Autodesk Inventor part; units mm, degrees
(part 2 of 3)
  line L885 (90.7927, 5.4708) -> (90.7927, 2.3716)
  line L886 (90.7927, 2.3716) -> (91.5937, 2.3716)
  line L887 (91.5937, 2.3716) -> (91.5937, 1.3712)
  line L888 (91.5937, 1.3712) -> (105.5927, 1.3712)
  line L889 (105.5927, 1.3712) -> (105.5927, 2.3716)
  line L890 (105.5927, 2.3716) -> (106.3937, 2.3716)
  line L891 (106.3937, 2.3716) -> (106.3937, 5.4708)
  line L892 (106.3937, 5.4708) -> (105.5927, 5.4708)
  line L893 (105.5927, 5.4708) -> (105.5927, 11.2708)
  line L894 (105.5927, 11.2708) -> (106.3937, 11.2708)
  line L895 (106.3937, 11.2708) -> (106.3937, 14.3714)
  line L896 (106.3937, 14.3714) -> (105.5927, 14.3714)
  line L897 (105.5927, 14.3714) -> (105.5927, 15.3705)
  line L898 (105.5927, 15.3705) -> (91.5937, 15.3705)
  line L899 (72.5437, 15.3705) -> (72.5437, 14.3714)
  line L900 (72.5437, 14.3714) -> (71.7427, 14.3714)
  line L901 (71.7427, 14.3714) -> (71.7427, 11.2708)
  line L902 (71.7427, 11.2708) -> (72.5437, 11.2708)
  line L903 (72.5437, 11.2708) -> (72.5437, 5.4708)
  line L904 (72.5437, 5.4708) -> (71.7427, 5.4708)
  line L905 (71.7427, 5.4708) -> (71.7427, 2.3716)
  line L906 (71.7427, 2.3716) -> (72.5437, 2.3716)
  line L907 (72.5437, 2.3716) -> (72.5437, 1.3712)
  line L908 (72.5437, 1.3712) -> (86.5427, 1.3712)
  line L909 (86.5427, 1.3712) -> (86.5427, 2.3716)
  line L910 (86.5427, 2.3716) -> (87.3437, 2.3716)
  line L911 (87.3437, 2.3716) -> (87.3437, 5.4708)
  line L912 (87.3437, 5.4708) -> (86.5427, 5.4708)
  line L913 (86.5427, 5.4708) -> (86.5427, 11.2708)
  line L914 (86.5427, 11.2708) -> (87.3437, 11.2708)
  line L915 (87.3437, 11.2708) -> (87.3437, 14.3714)
  line L916 (87.3437, 14.3714) -> (86.5427, 14.3714)
  line L917 (86.5427, 14.3714) -> (86.5427, 15.3705)
  line L918 (86.5427, 15.3705) -> (72.5437, 15.3705)
  line L919 (53.4937, 15.3705) -> (53.4937, 14.3714)
  line L920 (53.4937, 14.3714) -> (52.6927, 14.3714)
  line L921 (52.6927, 14.3714) -> (52.6927, 11.2708)
  line L922 (52.6927, 11.2708) -> (53.4937, 11.2708)
  line L923 (53.4937, 11.2708) -> (53.4937, 5.4708)
  line L924 (53.4937, 5.4708) -> (52.6927, 5.4708)
  line L925 (52.6927, 5.4708) -> (52.6927, 2.3716)
  line L926 (52.6927, 2.3716) -> (53.4937, 2.3716)
  line L927 (53.4937, 2.3716) -> (53.4937, 1.3712)
  line L928 (53.4937, 1.3712) -> (67.4927, 1.3712)
  line L929 (67.4927, 1.3712) -> (67.4927, 2.3716)
  line L930 (67.4927, 2.3716) -> (68.2937, 2.3716)
  line L931 (68.2937, 2.3716) -> (68.2937, 5.4708)
  line L932 (68.2937, 5.4708) -> (67.4927, 5.4708)
  line L933 (67.4927, 5.4708) -> (67.4927, 11.2708)
  line L934 (67.4927, 11.2708) -> (68.2937, 11.2708)
  line L935 (68.2937, 11.2708) -> (68.2937, 14.3714)
  line L936 (68.2937, 14.3714) -> (67.4927, 14.3714)
  line L937 (67.4927, 14.3714) -> (67.4927, 15.3705)
  line L938 (67.4927, 15.3705) -> (53.4937, 15.3705)
  line L939 (34.4437, 15.3705) -> (34.4437, 14.3714)
  line L940 (34.4437, 14.3714) -> (33.6427, 14.3714)
  line L941 (33.6427, 14.3714) -> (33.6427, 11.2708)
  line L942 (33.6427, 11.2708) -> (34.4437, 11.2708)
  line L943 (34.4437, 11.2708) -> (34.4437, 5.4708)
  line L944 (34.4437, 5.4708) -> (33.6427, 5.4708)
  line L945 (33.6427, 5.4708) -> (33.6427, 2.3716)
  line L946 (33.6427, 2.3716) -> (34.4437, 2.3716)
  line L947 (34.4437, 2.3716) -> (34.4437, 1.3712)
  line L948 (34.4437, 1.3712) -> (48.4427, 1.3712)
  line L949 (48.4427, 1.3712) -> (48.4427, 2.3716)
  line L950 (48.4427, 2.3716) -> (49.2437, 2.3716)
  line L951 (49.2437, 2.3716) -> (49.2437, 5.4708)
  line L952 (49.2437, 5.4708) -> (48.4427, 5.4708)
  line L953 (48.4427, 5.4708) -> (48.4427, 11.2708)
  line L954 (48.4427, 11.2708) -> (49.2437, 11.2708)
  line L955 (49.2437, 11.2708) -> (49.2437, 14.3714)
  line L956 (49.2437, 14.3714) -> (48.4427, 14.3714)
  line L957 (48.4427, 14.3714) -> (48.4427, 15.3705)
  line L958 (48.4427, 15.3705) -> (34.4437, 15.3705)
  line L959 (15.3937, 15.3705) -> (15.3937, 14.3714)
  line L960 (15.3937, 14.3714) -> (14.5927, 14.3714)
  line L961 (14.5927, 14.3714) -> (14.5927, 11.2708)
  line L962 (14.5927, 11.2708) -> (15.3937, 11.2708)
  line L963 (15.3937, 11.2708) -> (15.3937, 5.4708)
  line L964 (15.3937, 5.4708) -> (14.5927, 5.4708)
  line L965 (14.5927, 5.4708) -> (14.5927, 2.3716)
  line L966 (14.5927, 2.3716) -> (15.3937, 2.3716)
  line L967 (15.3937, 2.3716) -> (15.3937, 1.3712)
  line L968 (15.3937, 1.3712) -> (29.3927, 1.3712)
  line L969 (29.3927, 1.3712) -> (29.3927, 2.3716)
  line L970 (29.3927, 2.3716) -> (30.1937, 2.3716)
  line L971 (30.1937, 2.3716) -> (30.1937, 5.4708)
  line L972 (30.1937, 5.4708) -> (29.3927, 5.4708)
  line L973 (29.3927, 5.4708) -> (29.3927, 11.2708)
  line L974 (29.3927, 11.2708) -> (30.1937, 11.2708)
  line L975 (30.1937, 11.2708) -> (30.1937, 14.3714)
  line L976 (30.1937, 14.3714) -> (29.3927, 14.3714)
  line L977 (29.3927, 14.3714) -> (29.3927, 15.3705)
  line L978 (29.3927, 15.3705) -> (15.3937, 15.3705)
  line L979 (-3.6563, 15.3705) -> (-3.6563, 14.3714)
  line L980 (-3.6563, 14.3714) -> (-4.4573, 14.3714)
  line L981 (-4.4573, 14.3714) -> (-4.4573, 11.2708)
  line L982 (-4.4573, 11.2708) -> (-3.6563, 11.2708)
  line L983 (-3.6563, 11.2708) -> (-3.6563, 5.4708)
  line L984 (-3.6563, 5.4708) -> (-4.4573, 5.4708)
  line L985 (-4.4573, 5.4708) -> (-4.4573, 2.3716)
  line L986 (-4.4573, 2.3716) -> (-3.6563, 2.3716)
  line L987 (-3.6563, 2.3716) -> (-3.6563, 1.3712)
  line L988 (-3.6563, 1.3712) -> (10.3427, 1.3712)
  line L989 (10.3427, 1.3712) -> (10.3427, 2.3716)
  line L990 (10.3427, 2.3716) -> (11.1437, 2.3716)
  line L991 (11.1437, 2.3716) -> (11.1437, 5.4708)
  line L992 (11.1437, 5.4708) -> (10.3427, 5.4708)
  line L993 (10.3427, 5.4708) -> (10.3427, 11.2708)
  line L994 (10.3427, 11.2708) -> (11.1437, 11.2708)
  line L995 (11.1437, 11.2708) -> (11.1437, 14.3714)
  line L996 (11.1437, 14.3714) -> (10.3427, 14.3714)
  line L997 (10.3427, 14.3714) -> (10.3427, 15.3705)
  line L998 (10.3427, 15.3705) -> (-3.6563, 15.3705)
  line L999 (-22.7063, 15.3705) -> (-22.7063, 14.3714)
  line L1000 (-22.7063, 14.3714) -> (-23.5073, 14.3714)
  line L1001 (-23.5073, 14.3714) -> (-23.5073, 11.2708)
  line L1002 (-23.5073, 11.2708) -> (-22.7063, 11.2708)
  line L1003 (-22.7063, 11.2708) -> (-22.7063, 5.4708)
  line L1004 (-22.7063, 5.4708) -> (-23.5073, 5.4708)
  line L1005 (-23.5073, 5.4708) -> (-23.5073, 2.3716)
  line L1006 (-23.5073, 2.3716) -> (-22.7063, 2.3716)
  line L1007 (-22.7063, 2.3716) -> (-22.7063, 1.3712)
  line L1008 (-22.7063, 1.3712) -> (-8.7073, 1.3712)
  line L1009 (-8.7073, 1.3712) -> (-8.7073, 2.3716)
  line L1010 (-8.7073, 2.3716) -> (-7.9063, 2.3716)
  line L1011 (-7.9063, 2.3716) -> (-7.9063, 5.4708)
  line L1012 (-7.9063, 5.4708) -> (-8.7073, 5.4708)
  line L1013 (-8.7073, 5.4708) -> (-8.7073, 11.2708)
  line L1014 (-8.7073, 11.2708) -> (-7.9063, 11.2708)
  line L1015 (-7.9063, 11.2708) -> (-7.9063, 14.3714)
  line L1016 (-7.9063, 14.3714) -> (-8.7073, 14.3714)
  line L1017 (-8.7073, 14.3714) -> (-8.7073, 15.3705)
  line L1018 (-8.7073, 15.3705) -> (-22.7063, 15.3705)
  line L1019 (-41.7563, 15.3705) -> (-41.7563, 14.3714)
  line L1020 (-41.7563, 14.3714) -> (-42.5573, 14.3714)
  line L1021 (-42.5573, 14.3714) -> (-42.5573, 11.2708)
  line L1022 (-42.5573, 11.2708) -> (-41.7563, 11.2708)
  line L1023 (-41.7563, 11.2708) -> (-41.7563, 5.4708)
  line L1024 (-41.7563, 5.4708) -> (-42.5573, 5.4708)
  line L1025 (-42.5573, 5.4708) -> (-42.5573, 2.3716)
  line L1026 (-42.5573, 2.3716) -> (-41.7563, 2.3716)
  line L1027 (-41.7563, 2.3716) -> (-41.7563, 1.3712)
  line L1028 (-41.7563, 1.3712) -> (-27.7573, 1.3712)
  line L1029 (-27.7573, 1.3712) -> (-27.7573, 2.3716)
  line L1030 (-27.7573, 2.3716) -> (-26.9563, 2.3716)
  line L1031 (-26.9563, 2.3716) -> (-26.9563, 5.4708)
  line L1032 (-26.9563, 5.4708) -> (-27.7573, 5.4708)
  line L1033 (-27.7573, 5.4708) -> (-27.7573, 11.2708)
  line L1034 (-27.7573, 11.2708) -> (-26.9563, 11.2708)
  line L1035 (-26.9563, 11.2708) -> (-26.9563, 14.3714)
  line L1036 (-26.9563, 14.3714) -> (-27.7573, 14.3714)
  line L1037 (-27.7573, 14.3714) -> (-27.7573, 15.3705)
  line L1038 (-27.7573, 15.3705) -> (-41.7563, 15.3705)
  line L1039 (-60.8066, 15.3705) -> (-60.8066, 14.3714)
  line L1040 (-60.8066, 14.3714) -> (-61.6074, 14.3714)
  line L1041 (-61.6074, 14.3714) -> (-61.6074, 11.2708)
  line L1042 (-61.6074, 11.2708) -> (-60.8066, 11.2708)
  line L1043 (-60.8066, 11.2708) -> (-60.8066, 5.4708)
  line L1044 (-60.8066, 5.4708) -> (-61.6074, 5.4708)
  line L1045 (-61.6074, 5.4708) -> (-61.6074, 2.3716)
  line L1046 (-61.6074, 2.3716) -> (-60.8066, 2.3716)
  line L1047 (-60.8066, 2.3716) -> (-60.8066, 1.3712)
  line L1048 (-60.8066, 1.3712) -> (-46.8073, 1.3712)
  line L1049 (-46.8073, 1.3712) -> (-46.8073, 2.3716)
  line L1050 (-46.8073, 2.3716) -> (-46.0063, 2.3716)
  line L1051 (-46.0063, 2.3716) -> (-46.0063, 5.4708)
  line L1052 (-46.0063, 5.4708) -> (-46.8073, 5.4708)
  line L1053 (-46.8073, 5.4708) -> (-46.8073, 11.2708)
  line L1054 (-46.8073, 11.2708) -> (-46.0063, 11.2708)
  line L1055 (-46.0063, 11.2708) -> (-46.0063, 14.3714)
  line L1056 (-46.0063, 14.3714) -> (-46.8073, 14.3714)
  line L1057 (-46.8073, 14.3714) -> (-46.8073, 15.3705)
  line L1058 (-46.8073, 15.3705) -> (-60.8066, 15.3705)
  line L1059 (-79.8566, 15.3705) -> (-79.8566, 14.3714)
  line L1060 (-79.8566, 14.3714) -> (-80.6574, 14.3714)
  line L1061 (-80.6574, 14.3714) -> (-80.6574, 11.2708)
  line L1062 (-80.6574, 11.2708) -> (-79.8566, 11.2708)
  line L1063 (-79.8566, 11.2708) -> (-79.8566, 5.4708)
  line L1064 (-79.8566, 5.4708) -> (-80.6574, 5.4708)
  line L1065 (-80.6574, 5.4708) -> (-80.6574, 2.3716)
  line L1066 (-80.6574, 2.3716) -> (-79.8566, 2.3716)
  line L1067 (-79.8566, 2.3716) -> (-79.8566, 1.3712)
  line L1068 (-79.8566, 1.3712) -> (-65.8573, 1.3712)
  line L1069 (-65.8573, 1.3712) -> (-65.8573, 2.3716)
  line L1070 (-65.8573, 2.3716) -> (-65.0565, 2.3716)
  line L1071 (-65.0565, 2.3716) -> (-65.0565, 5.4708)
  line L1072 (-65.0565, 5.4708) -> (-65.8573, 5.4708)
  line L1073 (-65.8573, 5.4708) -> (-65.8573, 11.2708)
  line L1074 (-65.8573, 11.2708) -> (-65.0565, 11.2708)
  line L1075 (-65.0565, 11.2708) -> (-65.0565, 14.3714)
  line L1076 (-65.0565, 14.3714) -> (-65.8573, 14.3714)
  line L1077 (-65.8573, 14.3714) -> (-65.8573, 15.3705)
  line L1078 (-65.8573, 15.3705) -> (-79.8566, 15.3705)
  line L1079 (-98.9066, 15.3705) -> (-98.9066, 14.3714)
  line L1080 (-98.9066, 14.3714) -> (-99.7074, 14.3714)
  line L1081 (-99.7074, 14.3714) -> (-99.7074, 11.2708)
  line L1082 (-99.7074, 11.2708) -> (-98.9066, 11.2708)
  line L1083 (-98.9066, 11.2708) -> (-98.9066, 5.4708)
  line L1084 (-98.9066, 5.4708) -> (-99.7074, 5.4708)
  line L1085 (-99.7074, 5.4708) -> (-99.7074, 2.3716)
  line L1086 (-99.7074, 2.3716) -> (-98.9066, 2.3716)
  line L1087 (-98.9066, 2.3716) -> (-98.9066, 1.3712)
  line L1088 (-98.9066, 1.3712) -> (-84.9073, 1.3712)
  line L1089 (-84.9073, 1.3712) -> (-84.9073, 2.3716)
  line L1090 (-84.9073, 2.3716) -> (-84.1065, 2.3716)
  line L1091 (-84.1065, 2.3716) -> (-84.1065, 5.4708)
  line L1092 (-84.1065, 5.4708) -> (-84.9073, 5.4708)
  line L1093 (-84.9073, 5.4708) -> (-84.9073, 11.2708)
  line L1094 (-84.9073, 11.2708) -> (-84.1065, 11.2708)
  line L1095 (-84.1065, 11.2708) -> (-84.1065, 14.3714)
  line L1096 (-84.1065, 14.3714) -> (-84.9073, 14.3714)
  line L1097 (-84.9073, 14.3714) -> (-84.9073, 15.3705)
  line L1098 (-84.9073, 15.3705) -> (-98.9066, 15.3705)
  line L1099 (-117.9566, 15.3705) -> (-117.9566, 14.3714)
  line L1100 (-117.9566, 14.3714) -> (-118.7573, 14.3714)
  line L1101 (-118.7573, 14.3714) -> (-118.7573, 11.2708)
  line L1102 (-118.7573, 11.2708) -> (-117.9566, 11.2708)
  line L1103 (-117.9566, 11.2708) -> (-117.9566, 5.4708)
  line L1104 (-117.9566, 5.4708) -> (-118.7573, 5.4708)
  line L1105 (-118.7573, 5.4708) -> (-118.7573, 2.3716)
  line L1106 (-118.7573, 2.3716) -> (-117.9566, 2.3716)
  line L1107 (-117.9566, 2.3716) -> (-117.9566, 1.3712)
  line L1108 (-117.9566, 1.3712) -> (-103.9573, 1.3712)
  line L1109 (-103.9573, 1.3712) -> (-103.9573, 2.3716)
  line L1110 (-103.9573, 2.3716) -> (-103.1565, 2.3716)
  line L1111 (-103.1565, 2.3716) -> (-103.1565, 5.4708)
  line L1112 (-103.1565, 5.4708) -> (-103.9573, 5.4708)
  line L1113 (-103.9573, 5.4708) -> (-103.9573, 11.2708)
  line L1114 (-103.9573, 11.2708) -> (-103.1565, 11.2708)
  line L1115 (-103.1565, 11.2708) -> (-103.1565, 14.3714)
  line L1116 (-103.1565, 14.3714) -> (-103.9573, 14.3714)
  line L1117 (-103.9573, 14.3714) -> (-103.9573, 15.3705)
  line L1118 (-103.9573, 15.3705) -> (-117.9566, 15.3705)
  line L1119 (-141.7691, 15.3705) -> (-141.7691, 14.3714)
  line L1120 (-141.7691, 14.3714) -> (-142.5698, 14.3714)
  line L1121 (-142.5698, 14.3714) -> (-142.5698, 11.2708)
  line L1122 (-142.5698, 11.2708) -> (-141.7691, 11.2708)
  line L1123 (-141.7691, 11.2708) -> (-141.7691, 5.4708)
  line L1124 (-141.7691, 5.4708) -> (-142.5698, 5.4708)
  line L1125 (-142.5698, 5.4708) -> (-142.5698, 2.3716)
  line L1126 (-142.5698, 2.3716) -> (-141.7691, 2.3716)
  line L1127 (-141.7691, 2.3716) -> (-141.7691, 1.3712)
  line L1128 (-141.7691, 1.3712) -> (-127.7696, 1.3712)
  line L1129 (-127.7696, 1.3712) -> (-127.7696, 2.3716)
  line L1130 (-127.7696, 2.3716) -> (-126.9704, 2.3716)
  line L1131 (-126.9704, 2.3716) -> (-126.9704, 5.4708)
  line L1132 (-126.9704, 5.4708) -> (-127.7696, 5.4708)
  line L1133 (-127.7696, 5.4708) -> (-127.7696, 11.2708)
  line L1134 (-127.7696, 11.2708) -> (-126.9704, 11.2708)
  line L1135 (-126.9704, 11.2708) -> (-126.9704, 14.3714)
  line L1136 (-126.9704, 14.3714) -> (-127.7696, 14.3714)
  line L1137 (-127.7696, 14.3714) -> (-127.7696, 15.3705)
  line L1138 (-127.7696, 15.3705) -> (-141.7691, 15.3705)
  line L1139 (110.6437, 34.4205) -> (110.6437, 33.4214)
  line L1140 (110.6437, 33.4214) -> (109.8427, 33.4214)
  line L1141 (109.8427, 33.4214) -> (109.8427, 30.3208)
  line L1142 (109.8427, 30.3208) -> (110.6437, 30.3208)
  line L1143 (110.6437, 30.3208) -> (110.6437, 29.7214)
  line L1144 (110.6437, 29.7214) -> (109.1177, 29.7214)
  line L1145 (109.1177, 29.7214) -> (109.1177, 32.9515)
  line L1146 (109.1177, 32.9515) -> (102.3687, 32.9515)
  line L1147 (102.3687, 32.9515) -> (102.3687, 29.7214)
  line L1148 (102.3687, 29.7214) -> (101.5427, 29.7214)
  line L1149 (101.5427, 29.7214) -> (101.5427, 26.9211)
  line L1150 (101.5427, 26.9211) -> (102.3687, 26.9211)
  line L1151 (102.3687, 26.9211) -> (102.3687, 20.6512)
  line L1152 (102.3687, 20.6512) -> (104.0917, 20.6512)
  line L1153 (104.0917, 20.6512) -> (104.0917, 19.451)
  line L1154 (104.0917, 19.451) -> (107.3927, 19.451)
  line L1155 (107.3927, 19.451) -> (107.3927, 20.6512)
  line L1156 (107.3927, 20.6512) -> (109.1177, 20.6512)
  line L1157 (109.1177, 20.6512) -> (109.1177, 25.1216)
  line L1158 (109.1177, 25.1216) -> (110.6437, 25.1216)
  line L1159 (110.6437, 25.1216) -> (110.6437, 24.5208)
  line L1160 (110.6437, 24.5208) -> (109.8427, 24.5208)
  line L1161 (109.8427, 24.5208) -> (109.8427, 21.4216)
  line L1162 (109.8427, 21.4216) -> (110.6437, 21.4216)
  line L1163 (110.6437, 21.4216) -> (110.6437, 20.4212)
  line L1164 (110.6437, 20.4212) -> (124.6427, 20.4212)
  line L1165 (124.6427, 20.4212) -> (124.6427, 21.4216)
  line L1166 (124.6427, 21.4216) -> (125.4437, 21.4216)
  line L1167 (125.4437, 21.4216) -> (125.4437, 24.5208)
  line L1168 (125.4437, 24.5208) -> (124.6427, 24.5208)
  line L1169 (124.6427, 24.5208) -> (124.6427, 25.1216)
  line L1170 (124.6427, 25.1216) -> (126.1687, 25.1216)
  line L1171 (126.1687, 25.1216) -> (126.1687, 20.6512)
  line L1172 (126.1687, 20.6512) -> (127.8937, 20.6512)
  line L1173 (127.8937, 20.6512) -> (127.8937, 19.451)
  line L1174 (127.8937, 19.451) -> (131.1927, 19.451)
  line L1175 (131.1927, 19.451) -> (131.1927, 20.6512)
  line L1176 (131.1927, 20.6512) -> (132.9177, 20.6512)
  line L1177 (132.9177, 20.6512) -> (132.9177, 26.9211)
  line L1178 (132.9177, 26.9211) -> (133.7437, 26.9211)
  line L1179 (133.7437, 26.9211) -> (133.7437, 29.7214)
  line L1180 (133.7437, 29.7214) -> (132.9177, 29.7214)
  line L1181 (132.9177, 29.7214) -> (132.9177, 32.9515)
  line L1182 (132.9177, 32.9515) -> (126.1687, 32.9515)
  line L1183 (126.1687, 32.9515) -> (126.1687, 29.7214)
  line L1184 (126.1687, 29.7214) -> (124.6427, 29.7214)
  line L1185 (124.6427, 29.7214) -> (124.6427, 30.3208)
  line L1186 (124.6427, 30.3208) -> (125.4437, 30.3208)
  line L1187 (125.4437, 30.3208) -> (125.4437, 33.4214)
  line L1188 (125.4437, 33.4214) -> (124.6427, 33.4214)
  line L1189 (124.6427, 33.4214) -> (124.6427, 34.4205)
  line L1190 (124.6427, 34.4205) -> (110.6437, 34.4205)
  line L1191 (143.9807, 34.4205) -> (143.9807, 33.4214)
  line L1192 (143.9807, 33.4214) -> (143.1797, 33.4214)
  line L1193 (143.1797, 33.4214) -> (143.1797, 30.3208)
  line L1194 (143.1797, 30.3208) -> (143.9807, 30.3208)
  line L1195 (143.9807, 30.3208) -> (143.9807, 24.5208)
  line L1196 (143.9807, 24.5208) -> (143.1797, 24.5208)
  line L1197 (143.1797, 24.5208) -> (143.1797, 21.4216)
  line L1198 (143.1797, 21.4216) -> (143.9807, 21.4216)
  line L1199 (143.9807, 21.4216) -> (143.9807, 20.4212)
  line L1200 (143.9807, 20.4212) -> (157.9807, 20.4212)
  line L1201 (157.9807, 20.4212) -> (157.9807, 21.4216)
  line L1202 (157.9807, 21.4216) -> (158.7797, 21.4216)
  line L1203 (158.7797, 21.4216) -> (158.7797, 24.5208)
  line L1204 (158.7797, 24.5208) -> (157.9807, 24.5208)
  line L1205 (157.9807, 24.5208) -> (157.9807, 30.3208)
  line L1206 (157.9807, 30.3208) -> (158.7797, 30.3208)
  line L1207 (158.7797, 30.3208) -> (158.7797, 33.4214)
  line L1208 (158.7797, 33.4214) -> (157.9807, 33.4214)
  line L1209 (157.9807, 33.4214) -> (157.9807, 34.4205)
  line L1210 (157.9807, 34.4205) -> (143.9807, 34.4205)
  line L1211 (82.0687, 34.4205) -> (82.0687, 33.4214)
  line L1212 (82.0687, 33.4214) -> (81.2677, 33.4214)
  line L1213 (81.2677, 33.4214) -> (81.2677, 30.3208)
  line L1214 (81.2677, 30.3208) -> (82.0687, 30.3208)
  line L1215 (82.0687, 30.3208) -> (82.0687, 24.5208)
  line L1216 (82.0687, 24.5208) -> (81.2677, 24.5208)
  line L1217 (81.2677, 24.5208) -> (81.2677, 21.4216)
  line L1218 (81.2677, 21.4216) -> (82.0687, 21.4216)
  line L1219 (82.0687, 21.4216) -> (82.0687, 20.4212)
  line L1220 (82.0687, 20.4212) -> (96.0677, 20.4212)
  line L1221 (96.0677, 20.4212) -> (96.0677, 21.4216)
  line L1222 (96.0677, 21.4216) -> (96.8687, 21.4216)
  line L1223 (96.8687, 21.4216) -> (96.8687, 24.5208)
  line L1224 (96.8687, 24.5208) -> (96.0677, 24.5208)
  line L1225 (96.0677, 24.5208) -> (96.0677, 30.3208)
  line L1226 (96.0677, 30.3208) -> (96.8687, 30.3208)
  line L1227 (96.8687, 30.3208) -> (96.8687, 33.4214)
  line L1228 (96.8687, 33.4214) -> (96.0677, 33.4214)
  line L1229 (96.0677, 33.4214) -> (96.0677, 34.4205)
  line L1230 (96.0677, 34.4205) -> (82.0687, 34.4205)
  line L1231 (63.0187, 34.4205) -> (63.0187, 33.4214)
  line L1232 (63.0187, 33.4214) -> (62.2177, 33.4214)
  line L1233 (62.2177, 33.4214) -> (62.2177, 30.3208)
  line L1234 (62.2177, 30.3208) -> (63.0187, 30.3208)
  line L1235 (63.0187, 30.3208) -> (63.0187, 24.5208)
  line L1236 (63.0187, 24.5208) -> (62.2177, 24.5208)
  line L1237 (62.2177, 24.5208) -> (62.2177, 21.4216)
  line L1238 (62.2177, 21.4216) -> (63.0187, 21.4216)
  line L1239 (63.0187, 21.4216) -> (63.0187, 20.4212)
  line L1240 (63.0187, 20.4212) -> (77.0177, 20.4212)
  line L1241 (77.0177, 20.4212) -> (77.0177, 21.4216)
  line L1242 (77.0177, 21.4216) -> (77.8187, 21.4216)
  line L1243 (77.8187, 21.4216) -> (77.8187, 24.5208)
  line L1244 (77.8187, 24.5208) -> (77.0177, 24.5208)
  line L1245 (77.0177, 24.5208) -> (77.0177, 30.3208)
  line L1246 (77.0177, 30.3208) -> (77.8187, 30.3208)
  line L1247 (77.8187, 30.3208) -> (77.8187, 33.4214)
  line L1248 (77.8187, 33.4214) -> (77.0177, 33.4214)
  line L1249 (77.0177, 33.4214) -> (77.0177, 34.4205)
  line L1250 (77.0177, 34.4205) -> (63.0187, 34.4205)
  line L1251 (43.9687, 34.4205) -> (43.9687, 33.4214)
  line L1252 (43.9687, 33.4214) -> (43.1677, 33.4214)
  line L1253 (43.1677, 33.4214) -> (43.1677, 30.3208)
  line L1254 (43.1677, 30.3208) -> (43.9687, 30.3208)
  line L1255 (43.9687, 30.3208) -> (43.9687, 24.5208)
  line L1256 (43.9687, 24.5208) -> (43.1677, 24.5208)
  line L1257 (43.1677, 24.5208) -> (43.1677, 21.4216)
  line L1258 (43.1677, 21.4216) -> (43.9687, 21.4216)
  line L1259 (43.9687, 21.4216) -> (43.9687, 20.4212)
  line L1260 (43.9687, 20.4212) -> (57.9677, 20.4212)
  line L1261 (57.9677, 20.4212) -> (57.9677, 21.4216)
  line L1262 (57.9677, 21.4216) -> (58.7687, 21.4216)
  line L1263 (58.7687, 21.4216) -> (58.7687, 24.5208)
  line L1264 (58.7687, 24.5208) -> (57.9677, 24.5208)
  line L1265 (57.9677, 24.5208) -> (57.9677, 30.3208)
  line L1266 (57.9677, 30.3208) -> (58.7687, 30.3208)
  line L1267 (58.7687, 30.3208) -> (58.7687, 33.4214)
  line L1268 (58.7687, 33.4214) -> (57.9677, 33.4214)
  line L1269 (57.9677, 33.4214) -> (57.9677, 34.4205)
  line L1270 (57.9677, 34.4205) -> (43.9687, 34.4205)
  line L1271 (24.9187, 34.4205) -> (24.9187, 33.4214)
  line L1272 (24.9187, 33.4214) -> (24.1177, 33.4214)
  line L1273 (24.1177, 33.4214) -> (24.1177, 30.3208)
  line L1274 (24.1177, 30.3208) -> (24.9187, 30.3208)
  line L1275 (24.9187, 30.3208) -> (24.9187, 24.5208)
  line L1276 (24.9187, 24.5208) -> (24.1177, 24.5208)
  line L1277 (24.1177, 24.5208) -> (24.1177, 21.4216)
  line L1278 (24.1177, 21.4216) -> (24.9187, 21.4216)
  line L1279 (24.9187, 21.4216) -> (24.9187, 20.4212)
  line L1280 (24.9187, 20.4212) -> (38.9177, 20.4212)
  line L1281 (38.9177, 20.4212) -> (38.9177, 21.4216)
  line L1282 (38.9177, 21.4216) -> (39.7187, 21.4216)
  line L1283 (39.7187, 21.4216) -> (39.7187, 24.5208)
  line L1284 (39.7187, 24.5208) -> (38.9177, 24.5208)
  line L1285 (38.9177, 24.5208) -> (38.9177, 30.3208)
  line L1286 (38.9177, 30.3208) -> (39.7187, 30.3208)
  line L1287 (39.7187, 30.3208) -> (39.7187, 33.4214)
  line L1288 (39.7187, 33.4214) -> (38.9177, 33.4214)
  line L1289 (38.9177, 33.4214) -> (38.9177, 34.4205)
  line L1290 (38.9177, 34.4205) -> (24.9187, 34.4205)
  line L1291 (5.8687, 34.4205) -> (5.8687, 33.4214)
  line L1292 (5.8687, 33.4214) -> (5.0677, 33.4214)
  line L1293 (5.0677, 33.4214) -> (5.0677, 30.3208)
  line L1294 (5.0677, 30.3208) -> (5.8687, 30.3208)
  line L1295 (5.8687, 30.3208) -> (5.8687, 24.5208)
  line L1296 (5.8687, 24.5208) -> (5.0677, 24.5208)
  line L1297 (5.0677, 24.5208) -> (5.0677, 21.4216)
  line L1298 (5.0677, 21.4216) -> (5.8687, 21.4216)
  line L1299 (5.8687, 21.4216) -> (5.8687, 20.4212)
  line L1300 (5.8687, 20.4212) -> (19.8677, 20.4212)
  line L1301 (19.8677, 20.4212) -> (19.8677, 21.4216)
  line L1302 (19.8677, 21.4216) -> (20.6687, 21.4216)
  line L1303 (20.6687, 21.4216) -> (20.6687, 24.5208)
  line L1304 (20.6687, 24.5208) -> (19.8677, 24.5208)
  line L1305 (19.8677, 24.5208) -> (19.8677, 30.3208)
  line L1306 (19.8677, 30.3208) -> (20.6687, 30.3208)
  line L1307 (20.6687, 30.3208) -> (20.6687, 33.4214)
  line L1308 (20.6687, 33.4214) -> (19.8677, 33.4214)
  line L1309 (19.8677, 33.4214) -> (19.8677, 34.4205)
  line L1310 (19.8677, 34.4205) -> (5.8687, 34.4205)
  line L1311 (-13.1813, 34.4205) -> (-13.1813, 33.4214)
  line L1312 (-13.1813, 33.4214) -> (-13.9823, 33.4214)
  line L1313 (-13.9823, 33.4214) -> (-13.9823, 30.3208)
  line L1314 (-13.9823, 30.3208) -> (-13.1813, 30.3208)
  line L1315 (-13.1813, 30.3208) -> (-13.1813, 24.5208)
  line L1316 (-13.1813, 24.5208) -> (-13.9823, 24.5208)
  line L1317 (-13.9823, 24.5208) -> (-13.9823, 21.4216)
  line L1318 (-13.9823, 21.4216) -> (-13.1813, 21.4216)
  line L1319 (-13.1813, 21.4216) -> (-13.1813, 20.4212)
  line L1320 (-13.1813, 20.4212) -> (0.8177, 20.4212)
  line L1321 (0.8177, 20.4212) -> (0.8177, 21.4216)
  line L1322 (0.8177, 21.4216) -> (1.6187, 21.4216)
  line L1323 (1.6187, 21.4216) -> (1.6187, 24.5208)
  line L1324 (1.6187, 24.5208) -> (0.8177, 24.5208)
  line L1325 (0.8177, 24.5208) -> (0.8177, 30.3208)
  line L1326 (0.8177, 30.3208) -> (1.6187, 30.3208)
  line L1327 (1.6187, 30.3208) -> (1.6187, 33.4214)
  line L1328 (1.6187, 33.4214) -> (0.8177, 33.4214)
  line L1329 (0.8177, 33.4214) -> (0.8177, 34.4205)
  line L1330 (0.8177, 34.4205) -> (-13.1813, 34.4205)
  line L1331 (-32.2333, 34.4205) -> (-32.2333, 33.4214)
  line L1332 (-32.2333, 33.4214) -> (-33.0323, 33.4214)
  line L1333 (-33.0323, 33.4214) -> (-33.0323, 30.3208)
  line L1334 (-33.0323, 30.3208) -> (-32.2333, 30.3208)
  line L1335 (-32.2333, 30.3208) -> (-32.2333, 24.5208)
  line L1336 (-32.2333, 24.5208) -> (-33.0323, 24.5208)
  line L1337 (-33.0323, 24.5208) -> (-33.0323, 21.4216)
  line L1338 (-33.0323, 21.4216) -> (-32.2333, 21.4216)
  line L1339 (-32.2333, 21.4216) -> (-32.2333, 20.4212)
  line L1340 (-32.2333, 20.4212) -> (-18.2323, 20.4212)
  line L1341 (-18.2323, 20.4212) -> (-18.2323, 21.4216)
  line L1342 (-18.2323, 21.4216) -> (-17.4313, 21.4216)
  line L1343 (-17.4313, 21.4216) -> (-17.4313, 24.5208)
  line L1344 (-17.4313, 24.5208) -> (-18.2323, 24.5208)
  line L1345 (-18.2323, 24.5208) -> (-18.2323, 30.3208)
  line L1346 (-18.2323, 30.3208) -> (-17.4313, 30.3208)
  line L1347 (-17.4313, 30.3208) -> (-17.4313, 33.4214)
  line L1348 (-17.4313, 33.4214) -> (-18.2323, 33.4214)
  line L1349 (-18.2323, 33.4214) -> (-18.2323, 34.4205)
  line L1350 (-18.2323, 34.4205) -> (-32.2333, 34.4205)
  line L1351 (-51.283, 34.4205) -> (-51.283, 33.4214)
  line L1352 (-51.283, 33.4214) -> (-52.0824, 33.4214)
  line L1353 (-52.0824, 33.4214) -> (-52.0824, 30.3208)
  line L1354 (-52.0824, 30.3208) -> (-51.283, 30.3208)
  line L1355 (-51.283, 30.3208) -> (-51.283, 24.5208)
  line L1356 (-51.283, 24.5208) -> (-52.0824, 24.5208)
  line L1357 (-52.0824, 24.5208) -> (-52.0824, 21.4216)
  line L1358 (-52.0824, 21.4216) -> (-51.283, 21.4216)
  line L1359 (-51.283, 21.4216) -> (-51.283, 20.4212)
  line L1360 (-51.283, 20.4212) -> (-37.2823, 20.4212)
  line L1361 (-37.2823, 20.4212) -> (-37.2823, 21.4216)
  line L1362 (-37.2823, 21.4216) -> (-36.4833, 21.4216)
  line L1363 (-36.4833, 21.4216) -> (-36.4833, 24.5208)
  line L1364 (-36.4833, 24.5208) -> (-37.2823, 24.5208)
  line L1365 (-37.2823, 24.5208) -> (-37.2823, 30.3208)
  line L1366 (-37.2823, 30.3208) -> (-36.4833, 30.3208)
  line L1367 (-36.4833, 30.3208) -> (-36.4833, 33.4214)
  line L1368 (-36.4833, 33.4214) -> (-37.2823, 33.4214)
  line L1369 (-37.2823, 33.4214) -> (-37.2823, 34.4205)
  line L1370 (-37.2823, 34.4205) -> (-51.283, 34.4205)
  line L1371 (-70.3316, 34.4205) -> (-70.3316, 33.4214)
  line L1372 (-70.3316, 33.4214) -> (-71.1324, 33.4214)
  line L1373 (-71.1324, 33.4214) -> (-71.1324, 30.3208)
  line L1374 (-71.1324, 30.3208) -> (-70.3316, 30.3208)
  line L1375 (-70.3316, 30.3208) -> (-70.3316, 24.5208)
  line L1376 (-70.3316, 24.5208) -> (-71.1324, 24.5208)
  line L1377 (-71.1324, 24.5208) -> (-71.1324, 21.4216)
  line L1378 (-71.1324, 21.4216) -> (-70.3316, 21.4216)
  line L1379 (-70.3316, 21.4216) -> (-70.3316, 20.4212)
  line L1380 (-70.3316, 20.4212) -> (-56.3323, 20.4212)
  line L1381 (-56.3323, 20.4212) -> (-56.3323, 21.4216)
  line L1382 (-56.3323, 21.4216) -> (-55.5329, 21.4216)
  line L1383 (-55.5329, 21.4216) -> (-55.5329, 24.5208)
  line L1384 (-55.5329, 24.5208) -> (-56.3323, 24.5208)
  line L1385 (-56.3323, 24.5208) -> (-56.3323, 30.3208)
  line L1386 (-56.3323, 30.3208) -> (-55.5329, 30.3208)
  line L1387 (-55.5329, 30.3208) -> (-55.5329, 33.4214)
  line L1388 (-55.5329, 33.4214) -> (-56.3323, 33.4214)
  line L1389 (-56.3323, 33.4214) -> (-56.3323, 34.4205)
  line L1390 (-56.3323, 34.4205) -> (-70.3316, 34.4205)
  line L1391 (-89.3816, 34.4205) -> (-89.3816, 33.4214)
  line L1392 (-89.3816, 33.4214) -> (-90.1824, 33.4214)
  line L1393 (-90.1824, 33.4214) -> (-90.1824, 30.3208)
  line L1394 (-90.1824, 30.3208) -> (-89.3816, 30.3208)
  line L1395 (-89.3816, 30.3208) -> (-89.3816, 24.5208)
  line L1396 (-89.3816, 24.5208) -> (-90.1824, 24.5208)
  line L1397 (-90.1824, 24.5208) -> (-90.1824, 21.4216)
  line L1398 (-90.1824, 21.4216) -> (-89.3816, 21.4216)
  line L1399 (-89.3816, 21.4216) -> (-89.3816, 20.4212)
  line L1400 (-89.3816, 20.4212) -> (-75.3823, 20.4212)
  line L1401 (-75.3823, 20.4212) -> (-75.3823, 21.4216)
  line L1402 (-75.3823, 21.4216) -> (-74.5815, 21.4216)
  line L1403 (-74.5815, 21.4216) -> (-74.5815, 24.5208)
  line L1404 (-74.5815, 24.5208) -> (-75.3823, 24.5208)
  line L1405 (-75.3823, 24.5208) -> (-75.3823, 30.3208)
  line L1406 (-75.3823, 30.3208) -> (-74.5815, 30.3208)
  line L1407 (-74.5815, 30.3208) -> (-74.5815, 33.4214)
  line L1408 (-74.5815, 33.4214) -> (-75.3823, 33.4214)
  line L1409 (-75.3823, 33.4214) -> (-75.3823, 34.4205)
  line L1410 (-75.3823, 34.4205) -> (-89.3816, 34.4205)
  line L1411 (-108.4316, 34.4205) -> (-108.4316, 33.4214)
  line L1412 (-108.4316, 33.4214) -> (-109.2324, 33.4214)
  line L1413 (-109.2324, 33.4214) -> (-109.2324, 30.3208)
  line L1414 (-109.2324, 30.3208) -> (-108.4316, 30.3208)
  line L1415 (-108.4316, 30.3208) -> (-108.4316, 24.5208)
  line L1416 (-108.4316, 24.5208) -> (-109.2324, 24.5208)
  line L1417 (-109.2324, 24.5208) -> (-109.2324, 21.4216)
  line L1418 (-109.2324, 21.4216) -> (-108.4316, 21.4216)
  line L1419 (-108.4316, 21.4216) -> (-108.4316, 20.4212)
  line L1420 (-108.4316, 20.4212) -> (-94.4323, 20.4212)
  line L1421 (-94.4323, 20.4212) -> (-94.4323, 21.4216)
  line L1422 (-94.4323, 21.4216) -> (-93.6315, 21.4216)
  line L1423 (-93.6315, 21.4216) -> (-93.6315, 24.5208)
  line L1424 (-93.6315, 24.5208) -> (-94.4323, 24.5208)
  line L1425 (-94.4323, 24.5208) -> (-94.4323, 30.3208)
  line L1426 (-94.4323, 30.3208) -> (-93.6315, 30.3208)
  line L1427 (-93.6315, 30.3208) -> (-93.6315, 33.4214)
  line L1428 (-93.6315, 33.4214) -> (-94.4323, 33.4214)
  line L1429 (-94.4323, 33.4214) -> (-94.4323, 34.4205)
  line L1430 (-94.4323, 34.4205) -> (-108.4316, 34.4205)
  line L1431 (-127.4816, 34.4205) -> (-127.4816, 33.4214)
  line L1432 (-127.4816, 33.4214) -> (-128.2823, 33.4214)
  line L1433 (-128.2823, 33.4214) -> (-128.2823, 30.3208)
  line L1434 (-128.2823, 30.3208) -> (-127.4816, 30.3208)
  line L1435 (-127.4816, 30.3208) -> (-127.4816, 24.5208)
  line L1436 (-127.4816, 24.5208) -> (-128.2823, 24.5208)
  line L1437 (-128.2823, 24.5208) -> (-128.2823, 21.4216)
  line L1438 (-128.2823, 21.4216) -> (-127.4816, 21.4216)
  line L1439 (-127.4816, 21.4216) -> (-127.4816, 20.4212)
  line L1440 (-127.4816, 20.4212) -> (-113.4823, 20.4212)
  line L1441 (-113.4823, 20.4212) -> (-113.4823, 21.4216)
  line L1442 (-113.4823, 21.4216) -> (-112.6815, 21.4216)
  line L1443 (-112.6815, 21.4216) -> (-112.6815, 24.5208)
  line L1444 (-112.6815, 24.5208) -> (-113.4823, 24.5208)
  line L1445 (-113.4823, 24.5208) -> (-113.4823, 30.3208)
  line L1446 (-113.4823, 30.3208) -> (-112.6815, 30.3208)
  line L1447 (-112.6815, 30.3208) -> (-112.6815, 33.4214)
  line L1448 (-112.6815, 33.4214) -> (-113.4823, 33.4214)
  line L1449 (-113.4823, 33.4214) -> (-113.4823, 34.4205)
  line L1450 (-113.4823, 34.4205) -> (-127.4816, 34.4205)
  line L1451 (-146.5317, 34.4205) -> (-146.5317, 33.4214)
  line L1452 (-146.5317, 33.4214) -> (-147.3323, 33.4214)
  line L1453 (-147.3323, 33.4214) -> (-147.3323, 30.3208)
  line L1454 (-147.3323, 30.3208) -> (-146.5317, 30.3208)
  line L1455 (-146.5317, 30.3208) -> (-146.5317, 24.5208)
  line L1456 (-146.5317, 24.5208) -> (-147.3323, 24.5208)
  line L1457 (-147.3323, 24.5208) -> (-147.3323, 21.4216)
  line L1458 (-147.3323, 21.4216) -> (-146.5317, 21.4216)
  line L1459 (-146.5317, 21.4216) -> (-146.5317, 20.4212)
  line L1460 (-146.5317, 20.4212) -> (-132.5321, 20.4212)
  line L1461 (-132.5321, 20.4212) -> (-132.5321, 21.4216)
  line L1462 (-132.5321, 21.4216) -> (-131.7315, 21.4216)
  line L1463 (-131.7315, 21.4216) -> (-131.7315, 24.5208)
  line L1464 (-131.7315, 24.5208) -> (-132.5321, 24.5208)
  line L1465 (-132.5321, 24.5208) -> (-132.5321, 30.3208)
  line L1466 (-132.5321, 30.3208) -> (-131.7315, 30.3208)
  line L1467 (-131.7315, 30.3208) -> (-131.7315, 33.4214)
  line L1468 (-131.7315, 33.4214) -> (-132.5321, 33.4214)
  line L1469 (-132.5321, 33.4214) -> (-132.5321, 34.4205)
  line L1470 (-132.5321, 34.4205) -> (-146.5317, 34.4205)
  line L1471 (143.9807, 58.2329) -> (143.9807, 57.2329)
  line L1472 (143.9807, 57.2329) -> (143.1797, 57.2329)
  line L1473 (143.1797, 57.2329) -> (143.1797, 54.1329)
  line L1474 (143.1797, 54.1329) -> (143.9807, 54.1329)
  line L1475 (143.9807, 54.1329) -> (143.9807, 48.3329)
  line L1476 (143.9807, 48.3329) -> (143.1797, 48.3329)
  line L1477 (143.1797, 48.3329) -> (143.1797, 45.2329)
  line L1478 (143.1797, 45.2329) -> (143.9807, 45.2329)
  line L1479 (143.9807, 45.2329) -> (143.9807, 44.2339)
  line L1480 (143.9807, 44.2339) -> (157.9807, 44.2339)
  line L1481 (157.9807, 44.2339) -> (157.9807, 45.2329)
  line L1482 (157.9807, 45.2329) -> (158.7797, 45.2329)
  line L1483 (158.7797, 45.2329) -> (158.7797, 48.3329)
  line L1484 (158.7797, 48.3329) -> (157.9807, 48.3329)
  line L1485 (157.9807, 48.3329) -> (157.9807, 54.1329)
  line L1486 (157.9807, 54.1329) -> (158.7797, 54.1329)
  line L1487 (158.7797, 54.1329) -> (158.7797, 57.2329)
  line L1488 (158.7797, 57.2329) -> (157.9807, 57.2329)
  line L1489 (157.9807, 57.2329) -> (157.9807, 58.2329)
  line L1490 (157.9807, 58.2329) -> (143.9807, 58.2329)
  line L1491 (86.8307, 58.2329) -> (86.8307, 57.2329)
  line L1492 (86.8307, 57.2329) -> (86.0297, 57.2329)
  line L1493 (86.0297, 57.2329) -> (86.0297, 54.1329)
  line L1494 (86.0297, 54.1329) -> (86.8307, 54.1329)
  line L1495 (86.8307, 54.1329) -> (86.8307, 48.3329)
  line L1496 (86.8307, 48.3329) -> (86.0297, 48.3329)
  line L1497 (86.0297, 48.3329) -> (86.0297, 45.2329)
  line L1498 (86.0297, 45.2329) -> (86.8307, 45.2329)
  line L1499 (86.8307, 45.2329) -> (86.8307, 44.2339)
  line L1500 (86.8307, 44.2339) -> (100.8307, 44.2339)
  line L1501 (100.8307, 44.2339) -> (100.8307, 45.2329)
  line L1502 (100.8307, 45.2329) -> (101.6297, 45.2329)
  line L1503 (101.6297, 45.2329) -> (101.6297, 48.3329)
  line L1504 (101.6297, 48.3329) -> (100.8307, 48.3329)
  line L1505 (100.8307, 48.3329) -> (100.8307, 54.1329)
  line L1506 (100.8307, 54.1329) -> (101.6297, 54.1329)
  line L1507 (101.6297, 54.1329) -> (101.6297, 57.2329)
  line L1508 (101.6297, 57.2329) -> (100.8307, 57.2329)
  line L1509 (100.8307, 57.2329) -> (100.8307, 58.2329)
  line L1510 (100.8307, 58.2329) -> (86.8307, 58.2329)
  line L1511 (67.7807, 58.2329) -> (67.7807, 57.2329)
  line L1512 (67.7807, 57.2329) -> (66.9797, 57.2329)
  line L1513 (66.9797, 57.2329) -> (66.9797, 54.1329)
  line L1514 (66.9797, 54.1329) -> (67.7807, 54.1329)
  line L1515 (67.7807, 54.1329) -> (67.7807, 48.3329)
  line L1516 (67.7807, 48.3329) -> (66.9797, 48.3329)
  line L1517 (66.9797, 48.3329) -> (66.9797, 45.2329)
  line L1518 (66.9797, 45.2329) -> (67.7807, 45.2329)
  line L1519 (67.7807, 45.2329) -> (67.7807, 44.2339)
  line L1520 (67.7807, 44.2339) -> (81.7807, 44.2339)
  line L1521 (81.7807, 44.2339) -> (81.7807, 45.2329)
  line L1522 (81.7807, 45.2329) -> (82.5797, 45.2329)
  line L1523 (82.5797, 45.2329) -> (82.5797, 48.3329)
  line L1524 (82.5797, 48.3329) -> (81.7807, 48.3329)
  line L1525 (81.7807, 48.3329) -> (81.7807, 54.1329)
  line L1526 (81.7807, 54.1329) -> (82.5797, 54.1329)
  line L1527 (82.5797, 54.1329) -> (82.5797, 57.2329)
  line L1528 (82.5797, 57.2329) -> (81.7807, 57.2329)
  line L1529 (81.7807, 57.2329) -> (81.7807, 58.2329)
  line L1530 (81.7807, 58.2329) -> (67.7807, 58.2329)
  line L1531 (48.7307, 58.2329) -> (48.7307, 57.2329)
  line L1532 (48.7307, 57.2329) -> (47.9297, 57.2329)
  line L1533 (47.9297, 57.2329) -> (47.9297, 54.1329)
  line L1534 (47.9297, 54.1329) -> (48.7307, 54.1329)
  line L1535 (48.7307, 54.1329) -> (48.7307, 48.3329)
  line L1536 (48.7307, 48.3329) -> (47.9297, 48.3329)
  line L1537 (47.9297, 48.3329) -> (47.9297, 45.2329)
  line L1538 (47.9297, 45.2329) -> (48.7307, 45.2329)
  line L1539 (48.7307, 45.2329) -> (48.7307, 44.2339)
  line L1540 (48.7307, 44.2339) -> (62.7307, 44.2339)
  line L1541 (62.7307, 44.2339) -> (62.7307, 45.2329)
  line L1542 (62.7307, 45.2329) -> (63.5297, 45.2329)
  line L1543 (63.5297, 45.2329) -> (63.5297, 48.3329)
  line L1544 (63.5297, 48.3329) -> (62.7307, 48.3329)
  line L1545 (62.7307, 48.3329) -> (62.7307, 54.1329)
  line L1546 (62.7307, 54.1329) -> (63.5297, 54.1329)
  line L1547 (63.5297, 54.1329) -> (63.5297, 57.2329)
  line L1548 (63.5297, 57.2329) -> (62.7307, 57.2329)
  line L1549 (62.7307, 57.2329) -> (62.7307, 58.2329)
  line L1550 (62.7307, 58.2329) -> (48.7307, 58.2329)
  line L1551 (29.6807, 58.2329) -> (29.6807, 57.2329)
  line L1552 (29.6807, 57.2329) -> (28.8797, 57.2329)
  line L1553 (28.8797, 57.2329) -> (28.8797, 54.1329)
  line L1554 (28.8797, 54.1329) -> (29.6807, 54.1329)
  line L1555 (29.6807, 54.1329) -> (29.6807, 48.3329)
  line L1556 (29.6807, 48.3329) -> (28.8797, 48.3329)
  line L1557 (28.8797, 48.3329) -> (28.8797, 45.2329)
  line L1558 (28.8797, 45.2329) -> (29.6807, 45.2329)
  line L1559 (29.6807, 45.2329) -> (29.6807, 44.2339)
  line L1560 (29.6807, 44.2339) -> (43.6807, 44.2339)
  line L1561 (43.6807, 44.2339) -> (43.6807, 45.2329)
  line L1562 (43.6807, 45.2329) -> (44.4797, 45.2329)
  line L1563 (44.4797, 45.2329) -> (44.4797, 48.3329)
  line L1564 (44.4797, 48.3329) -> (43.6807, 48.3329)
  line L1565 (43.6807, 48.3329) -> (43.6807, 54.1329)
  line L1566 (43.6807, 54.1329) -> (44.4797, 54.1329)
  line L1567 (44.4797, 54.1329) -> (44.4797, 57.2329)
  line L1568 (44.4797, 57.2329) -> (43.6807, 57.2329)
  line L1569 (43.6807, 57.2329) -> (43.6807, 58.2329)
  line L1570 (43.6807, 58.2329) -> (29.6807, 58.2329)
  line L1571 (10.6307, 58.2329) -> (10.6307, 57.2329)
  line L1572 (10.6307, 57.2329) -> (9.8297, 57.2329)
  line L1573 (9.8297, 57.2329) -> (9.8297, 54.1329)
  line L1574 (9.8297, 54.1329) -> (10.6307, 54.1329)
  line L1575 (10.6307, 54.1329) -> (10.6307, 48.3329)
  line L1576 (10.6307, 48.3329) -> (9.8297, 48.3329)
  line L1577 (9.8297, 48.3329) -> (9.8297, 45.2329)
  line L1578 (9.8297, 45.2329) -> (10.6307, 45.2329)
  line L1579 (10.6307, 45.2329) -> (10.6307, 44.2339)
  line L1580 (10.6307, 44.2339) -> (24.6307, 44.2339)
  line L1581 (24.6307, 44.2339) -> (24.6307, 45.2329)
  line L1582 (24.6307, 45.2329) -> (25.4297, 45.2329)
  line L1583 (25.4297, 45.2329) -> (25.4297, 48.3329)
  line L1584 (25.4297, 48.3329) -> (24.6307, 48.3329)
  line L1585 (24.6307, 48.3329) -> (24.6307, 54.1329)
  line L1586 (24.6307, 54.1329) -> (25.4297, 54.1329)
  line L1587 (25.4297, 54.1329) -> (25.4297, 57.2329)
  line L1588 (25.4297, 57.2329) -> (24.6307, 57.2329)
  line L1589 (24.6307, 57.2329) -> (24.6307, 58.2329)
  line L1590 (24.6307, 58.2329) -> (10.6307, 58.2329)
  line L1591 (-8.4193, 58.2329) -> (-8.4193, 57.2329)
  line L1592 (-8.4193, 57.2329) -> (-9.2203, 57.2329)
  line L1593 (-9.2203, 57.2329) -> (-9.2203, 54.1329)
  line L1594 (-9.2203, 54.1329) -> (-8.4193, 54.1329)
  line L1595 (-8.4193, 54.1329) -> (-8.4193, 48.3329)
  line L1596 (-8.4193, 48.3329) -> (-9.2203, 48.3329)
  line L1597 (-9.2203, 48.3329) -> (-9.2203, 45.2329)
  line L1598 (-9.2203, 45.2329) -> (-8.4193, 45.2329)
  line L1599 (-8.4193, 45.2329) -> (-8.4193, 44.2339)
  line L1600 (-8.4193, 44.2339) -> (5.5807, 44.2339)
  line L1601 (5.5807, 44.2339) -> (5.5807, 45.2329)
  line L1602 (5.5807, 45.2329) -> (6.3797, 45.2329)
  line L1603 (6.3797, 45.2329) -> (6.3797, 48.3329)
  line L1604 (6.3797, 48.3329) -> (5.5807, 48.3329)
  line L1605 (5.5807, 48.3329) -> (5.5807, 54.1329)
  line L1606 (5.5807, 54.1329) -> (6.3797, 54.1329)
  line L1607 (6.3797, 54.1329) -> (6.3797, 57.2329)
  line L1608 (6.3797, 57.2329) -> (5.5807, 57.2329)
  line L1609 (5.5807, 57.2329) -> (5.5807, 58.2329)
  line L1610 (5.5807, 58.2329) -> (-8.4193, 58.2329)
  line L1611 (-27.4693, 58.2329) -> (-27.4693, 57.2329)
  line L1612 (-27.4693, 57.2329) -> (-28.2703, 57.2329)
  line L1613 (-28.2703, 57.2329) -> (-28.2703, 54.1329)
  line L1614 (-28.2703, 54.1329) -> (-27.4693, 54.1329)
  line L1615 (-27.4693, 54.1329) -> (-27.4693, 48.3329)
  line L1616 (-27.4693, 48.3329) -> (-28.2703, 48.3329)
  line L1617 (-28.2703, 48.3329) -> (-28.2703, 45.2329)
  line L1618 (-28.2703, 45.2329) -> (-27.4693, 45.2329)
  line L1619 (-27.4693, 45.2329) -> (-27.4693, 44.2339)
  line L1620 (-27.4693, 44.2339) -> (-13.4693, 44.2339)
  line L1621 (-13.4693, 44.2339) -> (-13.4693, 45.2329)
  line L1622 (-13.4693, 45.2329) -> (-12.6703, 45.2329)
  line L1623 (-12.6703, 45.2329) -> (-12.6703, 48.3329)
  line L1624 (-12.6703, 48.3329) -> (-13.4693, 48.3329)
  line L1625 (-13.4693, 48.3329) -> (-13.4693, 54.1329)
  line L1626 (-13.4693, 54.1329) -> (-12.6703, 54.1329)
  line L1627 (-12.6703, 54.1329) -> (-12.6703, 57.2329)
  line L1628 (-12.6703, 57.2329) -> (-13.4693, 57.2329)
  line L1629 (-13.4693, 57.2329) -> (-13.4693, 58.2329)
  line L1630 (-13.4693, 58.2329) -> (-27.4693, 58.2329)
  line L1631 (-46.5193, 58.2329) -> (-46.5193, 57.2329)
  line L1632 (-46.5193, 57.2329) -> (-47.3203, 57.2329)
  line L1633 (-47.3203, 57.2329) -> (-47.3203, 54.1329)
  line L1634 (-47.3203, 54.1329) -> (-46.5193, 54.1329)
  line L1635 (-46.5193, 54.1329) -> (-46.5193, 48.3329)
  line L1636 (-46.5193, 48.3329) -> (-47.3203, 48.3329)
  line L1637 (-47.3203, 48.3329) -> (-47.3203, 45.2329)
  line L1638 (-47.3203, 45.2329) -> (-46.5193, 45.2329)
  line L1639 (-46.5193, 45.2329) -> (-46.5193, 44.2339)
  line L1640 (-46.5193, 44.2339) -> (-32.5193, 44.2339)
  line L1641 (-32.5193, 44.2339) -> (-32.5193, 45.2329)
  line L1642 (-32.5193, 45.2329) -> (-31.7203, 45.2329)
  line L1643 (-31.7203, 45.2329) -> (-31.7203, 48.3329)
  line L1644 (-31.7203, 48.3329) -> (-32.5193, 48.3329)
  line L1645 (-32.5193, 48.3329) -> (-32.5193, 54.1329)
  line L1646 (-32.5193, 54.1329) -> (-31.7203, 54.1329)
  line L1647 (-31.7203, 54.1329) -> (-31.7203, 57.2329)
  line L1648 (-31.7203, 57.2329) -> (-32.5193, 57.2329)
  line L1649 (-32.5193, 57.2329) -> (-32.5193, 58.2329)
  line L1650 (-32.5193, 58.2329) -> (-46.5193, 58.2329)
  line L1651 (-65.5691, 58.2329) -> (-65.5691, 57.2329)
  line L1652 (-65.5691, 57.2329) -> (-66.3699, 57.2329)
  line L1653 (-66.3699, 57.2329) -> (-66.3699, 54.1329)
  line L1654 (-66.3699, 54.1329) -> (-65.5691, 54.1329)
  line L1655 (-65.5691, 54.1329) -> (-65.5691, 48.3329)
  line L1656 (-65.5691, 48.3329) -> (-66.3699, 48.3329)
  line L1657 (-66.3699, 48.3329) -> (-66.3699, 45.2329)
  line L1658 (-66.3699, 45.2329) -> (-65.5691, 45.2329)
  line L1659 (-65.5691, 45.2329) -> (-65.5691, 44.2339)
  line L1660 (-65.5691, 44.2339) -> (-51.5698, 44.2339)
  line L1661 (-51.5698, 44.2339) -> (-51.5698, 45.2329)
  line L1662 (-51.5698, 45.2329) -> (-50.7704, 45.2329)
  line L1663 (-50.7704, 45.2329) -> (-50.7704, 48.3329)
  line L1664 (-50.7704, 48.3329) -> (-51.5698, 48.3329)
  line L1665 (-51.5698, 48.3329) -> (-51.5698, 54.1329)
  line L1666 (-51.5698, 54.1329) -> (-50.7704, 54.1329)
  line L1667 (-50.7704, 54.1329) -> (-50.7704, 57.2329)
  line L1668 (-50.7704, 57.2329) -> (-51.5698, 57.2329)
  line L1669 (-51.5698, 57.2329) -> (-51.5698, 58.2329)
  line L1670 (-51.5698, 58.2329) -> (-65.5691, 58.2329)
  line L1671 (-84.6191, 58.2329) -> (-84.6191, 57.2329)
  line L1672 (-84.6191, 57.2329) -> (-85.4199, 57.2329)
  line L1673 (-85.4199, 57.2329) -> (-85.4199, 54.1329)
  line L1674 (-85.4199, 54.1329) -> (-84.6191, 54.1329)
  line L1675 (-84.6191, 54.1329) -> (-84.6191, 48.3329)
  line L1676 (-84.6191, 48.3329) -> (-85.4199, 48.3329)
  line L1677 (-85.4199, 48.3329) -> (-85.4199, 45.2329)
  line L1678 (-85.4199, 45.2329) -> (-84.6191, 45.2329)
  line L1679 (-84.6191, 45.2329) -> (-84.6191, 44.2339)
  line L1680 (-84.6191, 44.2339) -> (-70.6198, 44.2339)
  line L1681 (-70.6198, 44.2339) -> (-70.6198, 45.2329)
  line L1682 (-70.6198, 45.2329) -> (-69.8204, 45.2329)
  line L1683 (-69.8204, 45.2329) -> (-69.8204, 48.3329)
  line L1684 (-69.8204, 48.3329) -> (-70.6198, 48.3329)
  line L1685 (-70.6198, 48.3329) -> (-70.6198, 54.1329)
  line L1686 (-70.6198, 54.1329) -> (-69.8204, 54.1329)
  line L1687 (-69.8204, 54.1329) -> (-69.8204, 57.2329)
  line L1688 (-69.8204, 57.2329) -> (-70.6198, 57.2329)
  line L1689 (-70.6198, 57.2329) -> (-70.6198, 58.2329)
  line L1690 (-70.6198, 58.2329) -> (-84.6191, 58.2329)
  line L1691 (-103.6691, 58.2329) -> (-103.6691, 57.2329)
  line L1692 (-103.6691, 57.2329) -> (-104.4699, 57.2329)
  line L1693 (-104.4699, 57.2329) -> (-104.4699, 54.1329)
  line L1694 (-104.4699, 54.1329) -> (-103.6691, 54.1329)
  line L1695 (-103.6691, 54.1329) -> (-103.6691, 48.3329)
  line L1696 (-103.6691, 48.3329) -> (-104.4699, 48.3329)
  line L1697 (-104.4699, 48.3329) -> (-104.4699, 45.2329)
  line L1698 (-104.4699, 45.2329) -> (-103.6691, 45.2329)
  line L1699 (-103.6691, 45.2329) -> (-103.6691, 44.2339)
  line L1700 (-103.6691, 44.2339) -> (-89.6698, 44.2339)
  line L1701 (-89.6698, 44.2339) -> (-89.6698, 45.2329)
  line L1702 (-89.6698, 45.2329) -> (-88.8704, 45.2329)
  line L1703 (-88.8704, 45.2329) -> (-88.8704, 48.3329)
  line L1704 (-88.8704, 48.3329) -> (-89.6698, 48.3329)
  line L1705 (-89.6698, 48.3329) -> (-89.6698, 54.1329)
  line L1706 (-89.6698, 54.1329) -> (-88.8704, 54.1329)
  line L1707 (-88.8704, 54.1329) -> (-88.8704, 57.2329)
  line L1708 (-88.8704, 57.2329) -> (-89.6698, 57.2329)
  line L1709 (-89.6698, 57.2329) -> (-89.6698, 58.2329)
  line L1710 (-89.6698, 58.2329) -> (-103.6691, 58.2329)
  line L1711 (-122.7191, 58.2329) -> (-122.7191, 57.2329)
  line L1712 (-122.7191, 57.2329) -> (-123.5198, 57.2329)
  line L1713 (-123.5198, 57.2329) -> (-123.5198, 54.1329)
  line L1714 (-123.5198, 54.1329) -> (-122.7191, 54.1329)
  line L1715 (-122.7191, 54.1329) -> (-122.7191, 48.3329)
  line L1716 (-122.7191, 48.3329) -> (-123.5198, 48.3329)
  line L1717 (-123.5198, 48.3329) -> (-123.5198, 45.2329)
  line L1718 (-123.5198, 45.2329) -> (-122.7191, 45.2329)
  line L1719 (-122.7191, 45.2329) -> (-122.7191, 44.2339)
  line L1720 (-122.7191, 44.2339) -> (-108.7198, 44.2339)
  line L1721 (-108.7198, 44.2339) -> (-108.7198, 45.2329)
  line L1722 (-108.7198, 45.2329) -> (-107.9204, 45.2329)
  line L1723 (-107.9204, 45.2329) -> (-107.9204, 48.3329)
  line L1724 (-107.9204, 48.3329) -> (-108.7198, 48.3329)
  line L1725 (-108.7198, 48.3329) -> (-108.7198, 54.1329)
  line L1726 (-108.7198, 54.1329) -> (-107.9204, 54.1329)
  line L1727 (-107.9204, 54.1329) -> (-107.9204, 57.2329)
  line L1728 (-107.9204, 57.2329) -> (-108.7198, 57.2329)
  line L1729 (-108.7198, 57.2329) -> (-108.7198, 58.2329)
  line L1730 (-108.7198, 58.2329) -> (-122.7191, 58.2329)
  line L1731 (-146.5317, 58.2329) -> (-146.5317, 57.2329)
  line L1732 (-146.5317, 57.2329) -> (-147.3323, 57.2329)
  line L1733 (-147.3323, 57.2329) -> (-147.3323, 54.1329)
  line L1734 (-147.3323, 54.1329) -> (-146.5317, 54.1329)
  line L1735 (-146.5317, 54.1329) -> (-146.5317, 48.3329)
  line L1736 (-146.5317, 48.3329) -> (-147.3323, 48.3329)
  line L1737 (-147.3323, 48.3329) -> (-147.3323, 45.2329)
  line L1738 (-147.3323, 45.2329) -> (-146.5317, 45.2329)
  line L1739 (-146.5317, 45.2329) -> (-146.5317, 44.2339)
  line L1740 (-146.5317, 44.2339) -> (-132.5321, 44.2339)
  line L1741 (-132.5321, 44.2339) -> (-132.5321, 45.2329)
  line L1742 (-132.5321, 45.2329) -> (-131.7315, 45.2329)
  line L1743 (-131.7315, 45.2329) -> (-131.7315, 48.3329)
  line L1744 (-131.7315, 48.3329) -> (-132.5321, 48.3329)
  line L1745 (-132.5321, 48.3329) -> (-132.5321, 54.1329)
  line L1746 (-132.5321, 54.1329) -> (-131.7315, 54.1329)
  line L1747 (-131.7315, 54.1329) -> (-131.7315, 57.2329)
  line L1748 (-131.7315, 57.2329) -> (-132.5321, 57.2329)
  line L1749 (-132.5321, 57.2329) -> (-132.5321, 58.2329)
  line L1750 (-132.5321, 58.2329) -> (-146.5317, 58.2329)
  line L1751 (-152.0562, 60.7579) -> (-152.0562, 31.3429)
  line L1752 (-162.0562, -1.1571) -> (-162.0562, -26.1571)
  line L1753 (-162.0562, -1.1571) -> (-162.0562, 23.8429)
  line L1754 (-157.0562, -31.1571) -> (-154.5562, -31.1571)
  line L1755 (-157.0562, 28.8429) -> (-154.5562, 28.8429)
  line L1756 (-13.3822, 63.7581) -> (24.8087, 63.7581)
  line L1757 (160.4947, 63.7581) -> (89.8087, 63.7581)
  arc A0 (-157.0562, 28.8429) -> (-162.0562, 23.8429) centre (-157.0562, 23.8429) ccw
  arc A1 (-162.0562, -26.1571) -> (-157.0562, -31.1571) centre (-157.0562, -26.1571) ccw
  arc A2 (-152.0562, -33.6571) -> (-154.5562, -31.1571) centre (-154.5562, -33.6571) ccw
  arc A3 (-154.5562, 28.8429) -> (-152.0562, 31.3429) centre (-154.5562, 31.3429) ccw
  line L1758 (173.5067, -1.1571) -> (173.5067, 23.8429)
  line L1759 (173.5067, -1.1571) -> (173.5067, -26.1571)
  line L1760 (168.5067, 28.8429) -> (166.0067, 28.8429)
  line L1761 (168.5067, -31.1571) -> (166.0067, -31.1571)
  arc A4 (168.5067, -31.1571) -> (173.5067, -26.1571) centre (168.5067, -26.1571) ccw
  arc A5 (173.5067, 23.8429) -> (168.5067, 28.8429) centre (168.5067, 23.8429) ccw
  arc A6 (163.5067, 31.3429) -> (166.0067, 28.8429) centre (166.0067, 31.3429) ccw
  arc A7 (166.0067, -31.1571) -> (163.5067, -33.6571) centre (166.0067, -33.6571) ccw
  line L1762 (163.5067, -33.6571) -> (163.5067, -63.0674)
  line L1763 (-45.8822, 73.7581) -> (-70.8822, 73.7581)
  line L1764 (-45.8822, 73.7581) -> (-20.8822, 73.7581)
  line L1765 (-75.8822, 68.7581) -> (-75.8822, 66.2581)
  line L1766 (-15.8822, 68.7581) -> (-15.8822, 66.2581)
  arc A8 (-15.8822, 68.7581) -> (-20.8822, 73.7581) centre (-20.8822, 68.7581) ccw
  arc A9 (-70.8822, 73.7581) -> (-75.8822, 68.7581) centre (-70.8822, 68.7581) ccw
  arc A10 (-78.3822, 63.7581) -> (-75.8822, 66.2581) centre (-78.3822, 66.2581) ccw
  arc A11 (-15.8822, 66.2581) -> (-13.3822, 63.7581) centre (-13.3822, 66.2581) ccw
  line L1767 (57.3087, 73.7581) -> (32.3087, 73.7581)
  line L1768 (57.3087, 73.7581) -> (82.3087, 73.7581)
  line L1769 (27.3087, 68.7581) -> (27.3087, 66.2581)
  line L1770 (87.3087, 68.7581) -> (87.3087, 66.2581)
  arc A12 (87.3087, 68.7581) -> (82.3087, 73.7581) centre (82.3087, 68.7581) ccw